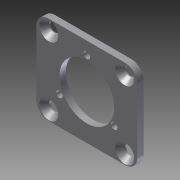
# Autodesk Inventor part: Dewalt Drill Cap Rotation plate
Saved by Autodesk Inventor 2012 (Build 160160000, 160)
## iProperties
Created: 2012-07-04
Part Number: Dewalt Drill Cap Rotation plate
Material: Default
Document SubType Name: Modeling
Designer: Bruce
Density: 1 g/cm^3
Author: Bruce
Autodesk Inventor part; units mm, degrees
ref_plane "YZ Plane" through (0, 0, 0) normal (1, 0, 0) x (0, 1, 0)
ref_plane "XZ Plane" through (0, 0, 0) normal (0, 1, 0) x (-1, 0, 0)
ref_plane "XY Plane" through (0, 0, 0) normal (0, 0, 1) x (1, 0, 0)
sketch "Sketch1" plane through (0, 0, 0) normal (0, 0, 1) x (1, 0, 0)
  line L0 (-31.75, 22.225) -> (31.75, 22.225)
  line L1 (31.75, 22.225) -> (31.75, -22.225)
  line L2 (31.75, -22.225) -> (-31.75, -22.225)
  line L3 (-31.75, -22.225) -> (-31.75, 22.225)
  circle A0 centre (0, 0) radius 13.716
  circle A1 centre (0, 0) radius 13.6017
  circle A2 centre (13.7482, -7.9375) radius 1.6193
  circle A3 centre (0, 0) radius 15.875 construction
  circle A4 centre (0, 15.875) radius 1.6193
  circle A5 centre (-13.7482, -7.9375) radius 1.6193
  circle A6 centre (0, 0) radius 21.59 construction
  line L4 (0, 0) -> (13.7482, -7.9375)
  line L5 (0, 0) -> (0, -22.225)
  line L6 (0, 0) -> (0, -22.225)
  line L7 (-31.75, 22.225) -> (-25.4, 22.225)
  line L8 (-25.4, 22.225) -> (-25.4, -22.225)
  line L9 (-25.4, -22.225) -> (-31.75, -22.225)
  line L10 (-31.75, -22.225) -> (-31.75, 22.225)
  line L11 (31.75, 22.225) -> (25.4, 22.225)
  line L12 (25.4, 22.225) -> (25.4, -22.225)
  line L13 (25.4, -22.225) -> (31.75, -22.225)
  line L14 (31.75, -22.225) -> (31.75, 22.225)
  point P0 (-19.05, 17.145)
  point P1 (-19.05, -17.145)
  point P2 (19.05, -17.145)
  point P3 (19.05, 17.145)
  dimension "d0" = 44.45
  dimension "d1" = 63.5
  dimension "d2" = 31.75
  dimension "d3" = 22.225
  dimension "d4" = 27.432
  dimension "d7" = 3.2385
  dimension "d9" = 15.875
  dimension "d15" = 360
  dimension "d17" = 43.18
  dimension "d18" = 5.08
  dimension "d19" = 5.08
  dimension "d20" = 19.05
  dimension "d21" = 19.05
  dimension "d31" = 34.29
  dimension "d32" = 38.1
  dimension "d35" = 60
  dimension "d36" = 6.35
  dimension "d37" = 6.35
  constraints: 30 end point, 7 equal length, 6 centre point, 4 coincident, 3 horizontal, 3 perpendicular, 2 horizontal alignment, 2 point on line, 2 vertical alignment, 1 midpoint, 10 other
  measures "d0" distance of L0.end L1.end
  measures "d1" distance of L1.end L2.end
  measures "d2" distance from line of L1 point (0, 0)
  measures "d3" distance from line of L2 point (0, 0)
  measures "d4" diameter of A0
  measures "d7" diameter of A2
  measures "d9" distance of A1.centre L4.end
  measures "d17" diameter of A6
  measures "d18" distance from line of point (-19.05, 17.145) L0
  measures "d19" distance from line of L2 point (-19.05, -17.145)
  measures "d20" horizontal distance of point (-19.05, -17.145) point (0, 0)
  measures "d21" horizontal distance of point (19.05, -17.145) point (0, 0)
  measures "d31" distance of point (-19.05, 17.145) point (-19.05, -17.145)
  measures "d32" distance of point (19.05, 17.145) point (-19.05, 17.145)
  measures "d35" angle of L6 L4
  measures "d36" distance between parallel lines of L8 L10
  measures "d37" distance between parallel lines of L14 L12
extrude "Extrusion1" add sketch "Sketch1" against normal blind 3.175
hole "Hole1" at (-19.05, 17.145, 0) at (-19.05, -17.145, 0) at (19.05, -17.145, 0) at (19.05, 17.145, 0) direction (0, 0, -1) diameter 4.9149 end through all countersink diameter 9.525 countersink angle 82
extrude "Extrusion2" cut sketch "Sketch1" against normal through all contours L0 L8 L2 L3 | L0 L1 L2 L12
fillet "Fillet1" radius 6.35 4 edges at (25.4, 22.225, -1.5875) (25.4, -22.225, -1.5875) (-25.4, -22.225, -1.5875) (-25.4, 22.225, -1.5875)
equation "\"d2\" = 0.5 * d1"
equation "\"d3\" = 0.5 * d0"
body "Solid1"
